Autodesk Fusion 360 part; units mm, degrees
note: some values were not read from the file. Set by a fixed rule: which sketch regions a step uses.
(part 3 of 4)
sketch "Sketch25" plane through (0, 0, 52.9247) normal (0, 0, 1) x (0, -1, 0)
  line L0 (-28.5, -58) -> (-28.5, -55)
  line L1 (-28.5, -58) -> (-25.5, -58)
  line L2 (-25.5, -58) -> (-25.5, -55)
  line L3 (-28.5, -55) -> (-33.0505, -55)
  line L4 (-25.5, -55) -> (-20.9495, -55)
  line L5 (-25.5, 81) -> (-28.5, 81)
  line L6 (-28.5, 81) -> (-28.5, 84)
  line L7 (-25.5, 81) -> (-25.5, 84)
  line L8 (-20.9495, 84) -> (-25.5, 84)
  line L9 (-28.5, 84) -> (-33.0505, 84)
  line L10 (-25.5, 43) -> (-28.5, 43)
  line L11 (-25.5, 46) -> (-28.5, 46)
  line L12 (-25.5, 43) -> (-25.5, 46)
  line L13 (-28.5, 46) -> (-28.5, 43)
  line L14 (-28.5, 56) -> (-25.5, 56)
  line L15 (-25.5, 56) -> (-25.5, 59)
  line L16 (-25.5, 59) -> (-28.5, 59)
  line L17 (-28.5, 59) -> (-28.5, 56)
  line L18 (-23.9495, 52.5) -> (-23.9495, 49.5)
  line L19 (-23.9495, 49.5) -> (-20.9495, 49.5)
  line L20 (-23.9495, 52.5) -> (-20.9495, 52.5)
  line L21 (-20.9495, -55) -> (-20.9495, 49.5)
  line L22 (-20.9495, 52.5) -> (-20.9495, 84)
  line L23 (-30.0505, 52.5) -> (-33.0505, 52.5)
  line L24 (-30.0505, 52.5) -> (-30.0505, 49.5)
  line L25 (-30.0505, 49.5) -> (-33.0505, 49.5)
  line L26 (-33.0505, -55) -> (-33.0505, 49.5)
  line L27 (-33.0505, 52.5) -> (-33.0505, 84)
  dimension "d397" = 139
  dimension "d398" = 139
  dimension "d432" = 12.1009
  dimension "d437" = 3
  dimension "d457" = 1.5505
  constraint coincident L0.end L3.start
  constraint perpendicular L0 L3
  constraint coincident L2.end L4.start
  constraint perpendicular L2 L4
  constraint perpendicular L3 L26
  constraint perpendicular L4 L21
  constraint horizontal L5
  constraint coincident L6.end L8
  constraint perpendicular L6 L8
  constraint perpendicular L7 L8
  constraint collinear L8 L9
  constraint horizontal L10
  constraint horizontal L11
  constraint perpendicular L11 L12
  constraint perpendicular L10 L13
  constraint perpendicular L14 L15
  constraint perpendicular L15 L16
  constraint collinear L21 L22
  constraint collinear L26 L27
  measures "d397" distance of L3.end L9.end
  measures "d398" distance of L4.end L8.start
  measures "d432" distance of L21 L26
  measures "d437" distance of L14.start L14.end
  measures "d457" horizontal distance of L14.end L18.start
extrude "Extrude53" add sketch "Sketch25" along normal blind 3 separate body makes body 53
ref_plane "WorkPlane25" through (81, 49.5, 28.7322) normal (1, 0, 0) x (0, 0, -1)
sketch "Sketch26" plane through (81, 0, 0) normal (1, 0, 0) x (0, 0, -1)
  line L0 (-46.9393, 8.4749) -> (-49.0607, 6.3536)
  line L1 (-49.0607, 6.3536) -> (-51.182, 8.4749)
  line L2 (-49.0607, 10.5962) -> (-51.182, 8.4749)
  line L3 (-49.0607, 10.5962) -> (-51.5355, 13.0711)
  line L4 (-51.9697, 15.5331) -> (-54.9241, 15.0121)
  line L5 (-54.9241, 15.0121) -> (-55.445, 17.9666)
  line L6 (-52.4906, 18.4875) -> (-55.445, 17.9666)
  line L7 (-52.9247, 20.9495) -> (-52.9247, 25.5)
  line L8 (-52.9247, 25.5) -> (-55.9247, 25.5)
  line L9 (-55.9247, 25.5) -> (-55.9247, 28.5)
  line L10 (-52.9247, 28.5) -> (-55.9247, 28.5)
  line L11 (-52.9247, 28.5) -> (-52.9247, 33.0505)
  line L12 (-52.4906, 35.5125) -> (-55.445, 36.0334)
  line L13 (-55.445, 36.0334) -> (-54.9241, 38.9879)
  line L14 (-51.9697, 38.4669) -> (-54.9241, 38.9879)
  line L15 (-51.5355, 40.9289) -> (-49.0607, 43.4038)
  line L16 (-49.0607, 43.4038) -> (-51.182, 45.5251)
  line L17 (-51.182, 45.5251) -> (-49.0607, 47.6464)
  line L18 (-46.9393, 45.5251) -> (-49.0607, 47.6464)
  line L19 (-44.4645, 6) -> (-30.2322, 6)
  line L20 (-30.2322, 6) -> (-30.2322, 3)
  line L21 (-27.2322, 3) -> (-30.2322, 3)
  line L22 (-27.2322, 6) -> (-27.2322, 3)
  line L23 (-27.2322, 6) -> (-13, 6)
  line L24 (-10, 25.5) -> (-13, 25.5)
  line L25 (-10, 28.5) -> (-10, 25.5)
  line L26 (-10, 28.5) -> (-13, 28.5)
  line L27 (-27.2322, 48) -> (-27.2322, 51)
  line L28 (-30.2322, 51) -> (-27.2322, 51)
  line L29 (-30.2322, 48) -> (-30.2322, 51)
  line L30 (-44.4645, 48) -> (-30.2322, 48)
  line L31 (-27.2322, 48) -> (-13, 48)
  line L32 (-13, 6) -> (-13, 25.5)
  line L33 (-13, 28.5) -> (-13, 48)
  line L34 (-44.4645, 6) -> (-46.9393, 8.4749)
  line L35 (-51.5355, 13.0711) -> (-51.9697, 15.5331)
  line L36 (-52.4906, 18.4875) -> (-52.9247, 20.9495)
  line L37 (-52.9247, 33.0505) -> (-52.4906, 35.5125)
  line L38 (-51.9697, 38.4669) -> (-51.5355, 40.9289)
  line L39 (-46.9393, 45.5251) -> (-44.4645, 48)
  line L40 (-32.9624, 28.5) -> (-32.9624, 25.5)
  line L41 (-32.9624, 25.5) -> (-35.9624, 25.5)
  line L42 (-32.9624, 28.5) -> (-35.9624, 28.5)
  line L43 (-35.9624, 28.5) -> (-35.9624, 25.5)
  line L44 (-42.4624, 25.5) -> (-42.4624, 28.5)
  line L45 (-42.4624, 25.5) -> (-45.4624, 25.5)
  line L46 (-45.4624, 25.5) -> (-45.4624, 28.5)
  line L47 (-45.4624, 28.5) -> (-42.4624, 28.5)
  dimension "d503" = 3
  dimension "d504" = 3
  dimension "d676" = 3
  dimension "d677" = 3
  constraint coincident L23.end L32.start
  constraint coincident L24.end L32.end
  constraint coincident L26.end L33.start
  constraint coincident L31.end L33.end
  constraint coincident L19.start L34.start
  constraint coincident L0.start L34.end
  constraint coincident L3.end L35.start
  constraint coincident L4.start L35.end
  constraint coincident L6.start L36.start
  constraint coincident L7.start L36.end
  constraint coincident L11.end L37.start
  constraint coincident L12.start L37.end
  constraint coincident L14.start L38.start
  constraint coincident L15.start L38.end
  constraint coincident L18.start L39.start
  constraint coincident L30.start L39.end
  constraint perpendicular L40 L41
  constraint perpendicular L40 L42
  constraint perpendicular L41 L43
  constraint vertical L44
  constraint perpendicular L44 L45
  constraint perpendicular L45 L46
  measures "d503" distance of L40.end L41.end
  measures "d504" distance of L40.start L42.end
  measures "d676" distance of L44.start L45.end
  measures "d677" distance of L45.end L46.end
extrude "Extrude54" add sketch "Sketch26" along normal blind 3 separate body makes body 54
ref_plane "WorkPlane26" through (84, 27, 32.9624) normal (1, 0, 0) x (0, 0, -1)
sketch "Sketch27" plane through (84, 0, 0) normal (1, 0, 0) x (0, 0, -1)
  line L0 (-35.9624, 28.5) -> (-32.9624, 28.5)
  line L1 (-35.9624, 25.5) -> (-32.9624, 25.5)
  line L2 (-32.9624, 25.5) -> (-32.9624, 28.5)
  line L3 (-35.9624, 28.5) -> (-35.9624, 25.5)
  circle A0 centre (-34.4812, 27) radius 21.4812
  line L4 (-42.4812, 25.5) -> (-42.4812, 28.5)
  line L5 (-42.4812, 25.5) -> (-45.4812, 25.5)
  line L6 (-45.4812, 25.5) -> (-45.4812, 28.5)
  line L7 (-45.4812, 28.5) -> (-42.4812, 28.5)
  dimension "d500" = 3
  dimension "d672" = 3
  dimension "d673" = 3
  dimension "d674" = 3
  constraint horizontal L0
  constraint perpendicular L0 L2
  constraint vertical L4
  constraint perpendicular L4 L5
  constraint perpendicular L5 L6
  measures "d500" distance of L0
  measures "d672" distance of L4.start L4.end
  measures "d673" distance of L4.start L5.end
  measures "d674" distance of L5.end L6.end
extrude "Extrude55" add sketch "Sketch27" along normal blind 3 separate body makes body 55
ref_plane "WorkPlane27" through (87, 27, 34.4812) normal (1, 0, 0) x (0, 0, -1)
sketch "Sketch28" plane through (87, 0, 0) normal (1, 0, 0) x (0, 0, -1)
  line L0 (-35.9624, 25.5) -> (-35.9624, 28.5)
  line L1 (-35.9624, 28.5) -> (-32.9624, 28.5)
  line L2 (-32.9624, 28.5) -> (-32.9624, 25.5)
  line L3 (-32.9624, 25.5) -> (-35.9624, 25.5)
  circle A0 centre (-34.4812, 27) radius 19.481
  line L4 (-42.4812, 25.5) -> (-42.4812, 28.5)
  line L5 (-42.4812, 25.5) -> (-45.4812, 25.5)
  line L6 (-45.4812, 25.5) -> (-45.4812, 28.5)
  line L7 (-45.4812, 28.5) -> (-42.4812, 28.5)
  line L8 (-42.4812, 28.5) -> (-42.4812, 25.5)
  line L9 (-42.4812, 25.5) -> (-45.4812, 25.5)
  line L10 (-45.4812, 25.5) -> (-45.4812, 28.5)
  line L11 (-45.4812, 28.5) -> (-42.4812, 28.5)
  dimension "d501" = 38.962
  dimension "d669" = 3
  dimension "d670" = 3
  constraint vertical L4
  constraint perpendicular L4 L5
  constraint perpendicular L5 L6
  measures "d501" diameter of A0
  measures "d669" distance of L4.start L5.end
  measures "d670" distance of L5.end L6.end
extrude "Extrude56" add sketch "Sketch28" along normal blind 3 separate body makes body 56
ref_plane "WorkPlane28" through (90, 27, 34.4812) normal (1, 0, 0) x (0, 0, -1)
sketch "Sketch29" plane through (90, 0, 0) normal (1, 0, 0) x (0, 0, -1)
  line L0 (-32.9624, 28.5) -> (-32.9624, 25.5)
  line L1 (-32.9624, 25.5) -> (-35.9624, 25.5)
  line L2 (-35.9624, 25.5) -> (-35.9624, 28.5)
  line L3 (-35.9624, 28.5) -> (-32.9624, 28.5)
  circle A0 centre (-34.4812, 27) radius 6
  line L4 (-42.4812, 28.5) -> (-42.4812, 25.5)
  line L5 (-42.4812, 25.5) -> (-45.4812, 25.5)
  line L6 (-45.4812, 25.5) -> (-45.4812, 28.5)
  line L7 (-45.4812, 28.5) -> (-42.4812, 28.5)
  dimension "d502" = 12
  measures "d502" diameter of A0
extrude "Extrude57" add sketch "Sketch29" along normal blind 3 separate body contours A0 makes body 57
ref_plane "WorkPlane29" through (51, 23.9495, 54.4247) normal (0, -1, 0) x (1, 0, 0)
sketch "Sketch30" plane through (0, 23.9495, 0) normal (0, -1, 0) x (1, 0, 0)
  line L0 (52.5, 52.9247) -> (49.5, 52.9247)
  line L1 (49.5, 52.9247) -> (49.5, 55.9247)
  line L2 (52.5, 52.9247) -> (52.5, 55.9247)
  line L3 (52.5, 55.9247) -> (59, 55.9247)
  line L4 (49.5, 55.9247) -> (43, 55.9247)
  line L5 (43, 55.9247) -> (43, 69.4247)
  line L6 (59, 55.9247) -> (59, 69.4247)
  line L7 (43, 69.4247) -> (46, 69.4247)
  line L8 (46, 69.4247) -> (46, 72.4247)
  line L9 (46, 72.4247) -> (43, 72.4247)
  line L10 (43, 72.4247) -> (43, 85.9247)
  line L11 (59, 69.4247) -> (56, 69.4247)
  line L12 (56, 69.4247) -> (56, 72.4247)
  line L13 (56, 72.4247) -> (59, 72.4247)
  line L14 (59, 72.4247) -> (59, 85.9247)
  line L15 (59, 85.9247) -> (43, 85.9247)
  dimension "d449" = 6.5
  dimension "d450" = 6.5
  dimension "d451" = 13.5
  dimension "d452" = 13.5
  dimension "d453" = 3
  dimension "d454" = 13.5
  dimension "d455" = 3
  dimension "d456" = 13.5
  constraint coincident L2.end L3.start
  constraint perpendicular L2 L3
  constraint coincident L1.end L4.start
  constraint perpendicular L1 L4
  constraint perpendicular L4 L5
  constraint perpendicular L3 L6
  constraint perpendicular L5 L7
  constraint perpendicular L7 L8
  constraint perpendicular L8 L9
  constraint perpendicular L9 L10
  constraint perpendicular L6 L11
  constraint perpendicular L11 L12
  constraint perpendicular L12 L13
  constraint perpendicular L13 L14
  measures "d449" distance of L1.end L4.end
  measures "d450" distance of L2.end L3.end
  measures "d451" distance of L4.end L5.end
  measures "d452" distance of L3.end L6.end
  measures "d453" distance of L7.end L8.end
  measures "d454" distance of L9.end L10.end
  measures "d455" distance of L11.end L12.end
  measures "d456" distance of L13.end L14.end
extrude "Extrude58" add sketch "Sketch30" along normal blind 3 separate body makes body 58
ref_plane "WorkPlane30" through (51, 30.0505, 54.4247) normal (0, 1, 0) x (-1, 0, 0)
sketch "Sketch31" plane through (0, 30.0505, 0) normal (0, 1, 0) x (-1, 0, 0)
  line L0 (-52.5, 55.9247) -> (-52.5, 52.9247)
  line L1 (-52.5, 52.9247) -> (-49.5, 52.9247)
  line L2 (-49.5, 52.9247) -> (-49.5, 55.9247)
  line L3 (-49.5, 55.9247) -> (-43, 55.9247)
  line L4 (-59, 55.9247) -> (-52.5, 55.9247)
  line L5 (-43, 55.9247) -> (-43, 69.4247)
  line L6 (-43, 69.4247) -> (-46, 69.4247)
  line L7 (-46, 69.4247) -> (-46, 72.4247)
  line L8 (-46, 72.4247) -> (-43, 72.4247)
  line L9 (-43, 72.4247) -> (-43, 85.9247)
  line L10 (-43, 85.9247) -> (-59, 85.9247)
  line L11 (-59, 85.9247) -> (-59, 72.4247)
  line L12 (-59, 72.4247) -> (-56, 72.4247)
  line L13 (-56, 72.4247) -> (-56, 69.4247)
  line L14 (-56, 69.4247) -> (-59, 69.4247)
  line L15 (-59, 69.4247) -> (-59, 55.9247)
extrude "Extrude59" add sketch "Sketch31" along normal blind 3 separate body makes body 59
ref_plane "WorkPlane31" through (56, 27, 54.4247) normal (1, 0, 0) x (0, 1, 0)
sketch "Sketch32" plane through (56, 0, 0) normal (1, 0, 0) x (0, 1, 0)
  line L0 (20.9495, 69.4247) -> (20.9495, 72.4247)
  line L1 (23.9495, 69.4247) -> (20.9495, 69.4247)
  line L2 (23.9495, 55.9247) -> (23.9495, 69.4247)
  line L3 (30.0505, 69.4247) -> (30.0505, 55.9247)
  line L4 (30.0505, 69.4247) -> (33.0505, 69.4247)
  line L5 (33.0505, 72.4247) -> (33.0505, 69.4247)
  line L6 (30.0505, 72.4247) -> (33.0505, 72.4247)
  line L7 (23.9495, 72.4247) -> (23.9495, 85.9247)
  line L8 (23.9495, 72.4247) -> (20.9495, 72.4247)
  line L9 (30.0505, 85.9247) -> (30.0505, 72.4247)
  line L10 (28.5, 52.9247) -> (28.5, 55.9247)
  line L11 (25.5, 52.9247) -> (28.5, 52.9247)
  line L12 (25.5, 52.9247) -> (25.5, 55.9247)
  line L13 (23.9495, 55.9247) -> (25.5, 55.9247)
  line L14 (28.5, 55.9247) -> (30.0505, 55.9247)
  line L15 (23.9495, 85.9247) -> (30.0505, 85.9247)
  constraint coincident L2.start L13.start
  constraint coincident L12.end L13.end
  constraint coincident L10.end L14.start
  constraint coincident L3.end L14.end
  constraint coincident L7.end L15.start
  constraint coincident L9.start L15.end
extrude "Extrude60" add sketch "Sketch32" along normal blind 3 separate body makes body 60
ref_plane "WorkPlane32" through (46, 27, 54.4247) normal (-1, 0, 0) x (0, -1, 0)
sketch "Sketch33" plane through (46, 0, 0) normal (-1, 0, 0) x (0, -1, 0)
  line L0 (-30.0505, 69.4247) -> (-33.0505, 69.4247)
  line L1 (-33.0505, 69.4247) -> (-33.0505, 72.4247)
  line L2 (-30.0505, 72.4247) -> (-33.0505, 72.4247)
  line L3 (-20.9495, 72.4247) -> (-20.9495, 69.4247)
  line L4 (-23.9495, 72.4247) -> (-20.9495, 72.4247)
  line L5 (-23.9495, 69.4247) -> (-20.9495, 69.4247)
  line L6 (-28.5, 52.9247) -> (-28.5, 55.9247)
  line L7 (-28.5, 52.9247) -> (-25.5, 52.9247)
  line L8 (-25.5, 52.9247) -> (-25.5, 55.9247)
  line L9 (-25.5, 55.9247) -> (-23.9495, 55.9247)
  line L10 (-28.5, 55.9247) -> (-30.0505, 55.9247)
  line L11 (-30.0505, 69.4247) -> (-30.0505, 55.9247)
  line L12 (-23.9495, 69.4247) -> (-23.9495, 55.9247)
  line L13 (-30.0505, 72.4247) -> (-30.0505, 85.9247)
  line L14 (-23.9495, 72.4247) -> (-23.9495, 85.9247)
  line L15 (-30.0505, 85.9247) -> (-23.9495, 85.9247)
  dimension "d462" = 1.5505
  dimension "d463" = 1.5505
  dimension "d464" = 13.5
  dimension "d465" = 13.5
  constraint coincident L8.end L9.start
  constraint perpendicular L8 L9
  constraint coincident L6.end L10.start
  constraint perpendicular L6 L10
  constraint coincident L0.start L11.start
  constraint coincident L5.start L12.start
  constraint coincident L2.start L13.start
  constraint perpendicular L2 L13
  constraint coincident L4.start L14.start
  constraint perpendicular L4 L14
  measures "d462" distance of L8.end L9.end
  measures "d463" distance of L6.end L10.end
  measures "d464" distance of L2.start L13.end
  measures "d465" distance of L4.start L14.end
extrude "Extrude61" add sketch "Sketch33" along normal blind 3 separate body makes body 61
ref_plane "WorkPlane33" through (51, 30.0505, 69.4247) normal (0, -1, 0) x (1, 0, 0)
sketch "Sketch34" plane through (0, 30.0505, 0) normal (0, -1, 0) x (1, 0, 0)
  line L0 (46, 55.9247) -> (56, 55.9247)
  line L1 (56, 55.9247) -> (56, 94.9247)
  line L2 (46, 55.9247) -> (46, 94.9247)
  line L3 (56, 94.9247) -> (46, 94.9247)
  point P0 (46, 55.9247)
  point P1 (56, 55.9247)
  dimension "d469" = 39
  dimension "d470" = 39
  constraint coincident P0 L0.start
  constraint coincident P1 L0.end
  constraint perpendicular L0 L1
  constraint perpendicular L0 L2
  measures "d469" distance of P1 L1.end
  measures "d470" distance of P0 L2.end
extrude "Extrude62" add sketch "Sketch34" along normal blind 3 separate body makes body 62
ref_plane "WorkPlane34" through (51, 27.0505, 75.4247) normal (0, -1, 0) x (0, 0, -1)
sketch "Sketch35" plane through (0, 27.0505, 0) normal (0, -1, 0) x (0, 0, -1)
  line L0 (-55.9247, 46) -> (-55.9247, 56)
  line L1 (-55.9247, 56) -> (-94.9247, 56)
  line L2 (-94.9247, 56) -> (-94.9247, 46)
  line L3 (-94.9247, 46) -> (-55.9247, 46)
extrude "Extrude63" add sketch "Sketch35" along normal blind 3 separate body makes body 63
ref_plane "WorkPlane35" through (51, 22.4495, 85.9247) normal (0, 0, 1) x (-1, 0, 0)
sketch "Sketch36" plane through (0, 0, 85.9247) normal (0, 0, 1) x (-1, 0, 0)
  line L0 (-56, -24.0505) -> (-46, -24.0505)
  line L1 (-46, -24.0505) -> (-46, -30.0505)
  line L2 (-46, -30.0505) -> (-56, -30.0505)
  line L3 (-56, -30.0505) -> (-56, -24.0505)
  line L4 (-63, -16.9495) -> (-38.8991, -16.9495)
  line L5 (-38.8991, -16.9495) -> (-38.8991, -37.0505)
  line L6 (-38.8991, -37.0505) -> (-63, -37.0505)
  line L7 (-63, -16.9495) -> (-63, -37.0505)
  point P0 (-56, -30.0505)
  point P1 (-56, -24.0505)
  point P2 (-46, -24.0505)
  point P3 (-46, -30.0505)
  point P4 (-63, -37.0505)
  dimension "d479" = 20.1009
  dimension "d480" = 24.1009
  dimension "d481" = 20.1009
  dimension "d483" = 24.1009
  constraint coincident P1 L0.start
  constraint coincident P2 L0.end
  constraint coincident P3 L1.end
  constraint coincident P0 L2.end
  constraint perpendicular L4 L5
  constraint coincident P4 L6.end
  measures "d479" distance of L4.start P4
  measures "d480" distance of L4.start L4.end
  measures "d481" distance of L4.end L5.end
  measures "d483" distance of L5.end P4
extrude "Extrude64" add sketch "Sketch36" along normal blind 3 separate body makes body 64
ref_plane "WorkPlane36" through (50.9495, 27, 88.9247) normal (0, 0, 1) x (1, 0, 0)
sketch "Sketch37" plane through (0, 0, 88.9247) normal (0, 0, 1) x (1, 0, 0)
  line L0 (46, 30.0505) -> (56, 30.0505)
  line L1 (56, 30.0505) -> (56, 24.0505)
  line L2 (56, 24.0505) -> (46, 24.0505)
  line L3 (46, 24.0505) -> (46, 30.0505)
  line L4 (38.8991, 16.9495) -> (63, 16.9495)
  line L5 (63, 16.9495) -> (63, 37.0505)
  line L6 (63, 37.0505) -> (38.8991, 37.0505)
  line L7 (38.8991, 37.0505) -> (38.8991, 16.9495)
extrude "Extrude65" add sketch "Sketch37" along normal blind 3 separate body makes body 65
ref_plane "WorkPlane37" through (50.9495, 27, 91.9247) normal (0, 0, 1) x (1, 0, 0)
sketch "Sketch38" plane through (0, 0, 91.9247) normal (0, 0, 1) x (1, 0, 0)
  line L0 (56, 24.0505) -> (46, 24.0505)
  line L1 (46, 24.0505) -> (46, 30.0505)
  line L2 (46, 30.0505) -> (56, 30.0505)
  line L3 (56, 30.0505) -> (56, 24.0505)
  line L4 (38.8991, 37.0505) -> (38.8991, 16.9495)
  line L5 (38.8991, 16.9495) -> (63, 16.9495)
  line L6 (63, 16.9495) -> (63, 37.0505)
  line L7 (63, 37.0505) -> (38.8991, 37.0505)
extrude "Extrude66" add sketch "Sketch38" along normal blind 3 separate body makes body 66
ref_plane "WorkPlane38" through (87.0475, -8.5221, 11.5) normal (0.643192, -0.765705, 0) x (0.765705, 0.643192, 0)
sketch "Sketch39" plane through (40.2083, -47.867, 0) normal (0.643192, -0.765705, 0) x (0.765705, 0.643192, 0)
  line L0 (59.6713, 10) -> (59.6713, 13)
  line L1 (59.6713, 13) -> (62.6713, 13)
  line L2 (62.6713, 10) -> (89.821, 10)
  line L3 (62.6713, 10) -> (62.6713, 13)
  line L4 (89.821, 10) -> (89.821, 13)
  line L5 (89.821, 13) -> (92.821, 13)
  line L6 (92.821, 10) -> (111.9706, 10)
  line L7 (111.9706, 10) -> (111.9706, 13)
  line L8 (111.9706, 13) -> (114.9706, 13)
  line L9 (92.821, 10) -> (92.821, 13)
  line L10 (56.6713, 8) -> (56.6713, -10)
  line L11 (112.9703, -10) -> (112.9703, 8)
  line L12 (59.6344, 8) -> (59.6344, -10)
  line L13 (62.5975, 8) -> (62.5975, -10)
  line L14 (65.5606, 8) -> (65.5606, -10)
  line L15 (68.5238, 8) -> (68.5238, -10)
  line L16 (71.4869, 8) -> (71.4869, -10)
  line L17 (74.45, 8) -> (74.45, -10)
  line L18 (77.4131, 8) -> (77.4131, -10)
  line L19 (80.3762, 8) -> (80.3762, -10)
  line L20 (83.3393, 8) -> (83.3393, -10)
  line L21 (86.3024, 8) -> (86.3024, -10)
  line L22 (89.2655, 8) -> (89.2655, -10)
  line L23 (92.2286, 8) -> (92.2286, -10)
  line L24 (95.1917, 8) -> (95.1917, -10)
  line L25 (98.1548, 8) -> (98.1548, -10)
  line L26 (101.1179, 8) -> (101.1179, -10)
  line L27 (104.081, 8) -> (104.081, -10)
  line L28 (107.0441, 8) -> (107.0441, -10)
  line L29 (110.0072, 8) -> (110.0072, -10)
  line L30 (112.9703, 8) -> (112.9703, -10)
  line L31 (56.6713, 8) -> (59.6344, 8)
  line L32 (62.5975, 8) -> (65.5606, 8)
  line L33 (68.5238, 8) -> (71.4869, 8)
  line L34 (74.45, 8) -> (77.4131, 8)
  line L35 (80.3762, 8) -> (83.3393, 8)
  line L36 (86.3024, 8) -> (89.2655, 8)
  line L37 (92.2286, 8) -> (95.1917, 8)
  line L38 (98.1548, 8) -> (101.1179, 8)
  line L39 (104.081, 8) -> (107.0441, 8)
  line L40 (110.0072, 8) -> (112.9703, 8)
  line L41 (115.9706, 10) -> (115.9706, -12)
  line L42 (114.9706, 13) -> (114.9706, 10)
  line L43 (114.9706, 10) -> (115.9706, 10)
  line L44 (53.6713, 10) -> (53.6713, -12)
  line L45 (59.6713, 10) -> (53.6713, 10)
  line L46 (59.6344, -10) -> (56.6713, -10)
  line L47 (65.5606, -10) -> (62.5975, -10)
  line L48 (71.4869, -10) -> (68.5238, -10)
  line L49 (77.4131, -10) -> (74.45, -10)
  line L50 (83.3393, -10) -> (80.3762, -10)
  line L51 (89.2655, -10) -> (86.3024, -10)
  line L52 (95.1917, -10) -> (92.2286, -10)
  line L53 (101.1179, -10) -> (98.1548, -10)
  line L54 (112.9703, -10) -> (110.0072, -10)
  line L55 (107.0441, -10) -> (104.081, -10)
  line L56 (115.9706, -12) -> (53.6713, -12)
  dimension "d547" = 56.299
  constraint vertical L10
  constraint collinear L31 L32
  constraint collinear L32 L33
  constraint collinear L33 L34
  constraint collinear L34 L35
  constraint collinear L35 L36
  constraint collinear L36 L37
  constraint collinear L37 L38
  constraint collinear L38 L39
  constraint collinear L39 L40
  constraint coincident L8.end L42.start
  constraint perpendicular L8 L42
  constraint perpendicular L41 L43
  constraint coincident L0.start L45.start
  constraint perpendicular L44 L45
  constraint coincident L12.end L54
  constraint collinear L46 L54
  constraint coincident L14.end L54
  constraint collinear L47 L54
  constraint coincident L16.end L54
  constraint collinear L48 L54
  constraint coincident L18.end L54
  constraint collinear L49 L54
  constraint coincident L20.end L54
  constraint collinear L50 L54
  constraint coincident L22.end L54
  constraint collinear L51 L54
  constraint coincident L24.end L54
  constraint collinear L52 L54
  constraint coincident L26.end L54
  constraint collinear L53 L54
  constraint coincident L28.end L54
  constraint collinear L54 L55
  measures "d547" distance of L10.start L11.end
extrude "Extrude67" add sketch "Sketch39" along normal blind 3 separate body makes body 67
ref_plane "WorkPlane39" through (87.0475, 62.5221, 11.5) normal (0.643192, 0.765705, 0) x (-0.765705, 0.643192, 0)
sketch "Sketch40" plane through (66.8031, 79.5275, 0) normal (0.643192, 0.765705, 0) x (-0.765705, 0.643192, 0)
  line L0 (-27.939, 10) -> (-27.939, 13)
  line L1 (-27.939, 13) -> (-24.939, 13)
  line L2 (-27.939, 10) -> (-55.0886, 10)
  line L3 (-24.939, 10) -> (-24.939, 13)
  line L4 (-55.0886, 10) -> (-55.0886, 13)
  line L5 (-58.0886, 13) -> (-55.0886, 13)
  line L6 (-58.0886, 10) -> (-77.2383, 10)
  line L7 (-77.2383, 10) -> (-77.2383, 13)
  line L8 (-80.2383, 13) -> (-77.2383, 13)
  line L9 (-58.0886, 10) -> (-58.0886, 13)
  line L10 (-80.2383, 10) -> (-80.2383, 13)
  line L11 (-21.939, 8) -> (-21.939, -10)
  line L12 (-78.2383, 8) -> (-78.2383, -10)
  line L13 (-24.9021, 8) -> (-24.9021, -10)
  line L14 (-27.8652, 8) -> (-27.8652, -10)
  line L15 (-30.8283, 8) -> (-30.8283, -10)
  line L16 (-33.7914, 8) -> (-33.7914, -10)
  line L17 (-36.7546, 8) -> (-36.7546, -10)
  line L18 (-39.7177, 8) -> (-39.7177, -10)
  line L19 (-42.6808, 8) -> (-42.6808, -10)
  line L20 (-45.6439, 8) -> (-45.6439, -10)
  line L21 (-48.6071, 8) -> (-48.6071, -10)
  line L22 (-51.5702, 8) -> (-51.5702, -10)
  line L23 (-54.5333, 8) -> (-54.5333, -10)
  line L24 (-57.4964, 8) -> (-57.4964, -10)
  line L25 (-60.4595, 8) -> (-60.4595, -10)
  line L26 (-63.4227, 8) -> (-63.4227, -10)
  line L27 (-66.3858, 8) -> (-66.3858, -10)
  line L28 (-69.3489, 8) -> (-69.3489, -10)
  line L29 (-72.312, 8) -> (-72.312, -10)
  line L30 (-75.2751, 8) -> (-75.2751, -10)
  line L31 (-78.2383, 8) -> (-78.2383, -10)
  line L32 (-21.939, 8) -> (-24.9021, 8)
  line L33 (-27.8652, 8) -> (-30.8283, 8)
  line L34 (-33.7914, 8) -> (-36.7546, 8)
  line L35 (-39.7177, 8) -> (-42.6808, 8)
  line L36 (-45.6439, 8) -> (-48.6071, 8)
  line L37 (-51.5702, 8) -> (-54.5333, 8)
  line L38 (-57.4964, 8) -> (-60.4595, 8)
  line L39 (-63.4227, 8) -> (-66.3858, 8)
  line L40 (-69.3489, 8) -> (-72.312, 8)
  line L41 (-75.2751, 8) -> (-78.2383, 8)
  line L42 (-81.2383, 10) -> (-81.2383, -12)
  line L43 (-81.2383, 10) -> (-80.2383, 10)
  line L44 (-18.939, 10) -> (-18.939, -12)
  line L45 (-24.939, 10) -> (-18.939, 10)
  line L46 (-24.9021, -10) -> (-21.939, -10)
  line L47 (-30.8283, -10) -> (-27.8652, -10)
  line L48 (-36.7546, -10) -> (-33.7914, -10)
  line L49 (-42.6808, -10) -> (-39.7177, -10)
  line L50 (-48.6071, -10) -> (-45.6439, -10)
  line L51 (-54.5333, -10) -> (-51.5702, -10)
  line L52 (-60.4595, -10) -> (-57.4964, -10)
  line L53 (-66.3858, -10) -> (-63.4227, -10)
  line L54 (-72.312, -10) -> (-69.3489, -10)
  line L55 (-78.2383, -10) -> (-75.2751, -10)
  line L56 (-81.2383, -12) -> (-18.939, -12)
  constraint perpendicular L11 L32
  constraint collinear L32 L33
  constraint collinear L33 L34
  constraint collinear L34 L35
  constraint collinear L35 L36
  constraint collinear L36 L37
  constraint collinear L37 L38
  constraint collinear L38 L39
  constraint collinear L39 L40
  constraint collinear L40 L41
  constraint coincident L10.start L43.end
  constraint perpendicular L10 L43
  constraint coincident L3.start L45.start
  constraint perpendicular L44 L45
extrude "Extrude68" add sketch "Sketch40" along normal blind 3 separate body makes body 68
ref_plane "WorkPlane40" through (90, 27, 34.4812) normal (1, 0, 0) x (0, 0, -1)
sketch "Sketch41" plane through (90, 0, 0) normal (1, 0, 0) x (0, 0, -1)
  arc A0 (-34.4812, 34) -> (-34.4812, 20) centre (-34.4812, 27) ccw
  arc A1 (-34.4812, 39) -> (-34.4812, 15) centre (-34.4812, 27) ccw
  line L0 (-34.4812, 34) -> (-34.4812, 39)
  line L1 (-34.4812, 20) -> (-34.4812, 15)
  line L2 (-45.4812, 25.5) -> (-42.4812, 25.5)
  line L3 (-42.4812, 28.5) -> (-45.4812, 28.5)
  line L4 (-45.4812, 25.5) -> (-45.4812, 28.5)
  line L5 (-42.4812, 28.5) -> (-42.4812, 25.5)
  dimension "d594" = 3
  dimension "d595" = 3
  constraint vertical L0
  constraint parallel L0 L1
  constraint parallel L4 L5
  measures "d594" distance of L2.start L2.end
  measures "d595" distance of L3.start L3.end
extrude "Extrude69" add sketch "Sketch41" along normal blind 3 separate body makes body 69
ref_plane "WorkPlane41" through (93, 27, 40.4812) normal (1, 0, 0) x (0, 0, -1)
sketch "Sketch42" plane through (93, 0, 0) normal (1, 0, 0) x (0, 0, -1)
  line L0 (-42.4812, 25.5) -> (-45.4812, 25.5)
  line L1 (-45.4812, 25.5) -> (-45.4812, 28.5)
  line L2 (-45.4812, 28.5) -> (-42.4812, 28.5)
  line L3 (-42.4812, 28.5) -> (-42.4812, 25.5)
  line L4 (-34.4812, 34) -> (-34.4812, 39)
  arc A0 (-34.4812, 39) -> (-34.4812, 15) centre (-34.4812, 27) ccw
  line L5 (-34.4812, 15) -> (-34.4812, 20)
  arc A1 (-34.4812, 34) -> (-34.4812, 20) centre (-34.4812, 27) ccw
extrude "Extrude70" add sketch "Sketch42" along normal blind 3 separate body makes body 70
ref_plane "WorkPlane42" through (96, 27, 40.4812) normal (1, 0, 0) x (0, 0, -1)
sketch "Sketch43" plane through (96, 0, 0) normal (1, 0, 0) x (0, 0, -1)
  line L0 (-45.4812, 28.5) -> (-42.4812, 28.5)
  line L1 (-42.4812, 28.5) -> (-42.4812, 25.5)
  line L2 (-42.4812, 25.5) -> (-45.4812, 25.5)
  line L3 (-45.4812, 25.5) -> (-45.4812, 28.5)
  arc A0 (-34.4812, 39) -> (-34.4812, 15) centre (-34.4812, 27) ccw
  line L4 (-34.4812, 15) -> (-34.4812, 20)
  arc A1 (-34.4812, 34) -> (-34.4812, 20) centre (-34.4812, 27) ccw
  line L5 (-34.4812, 34) -> (-34.4812, 39)
extrude "Extrude71" add sketch "Sketch43" along normal blind 3 separate body makes body 71
ref_plane "WorkPlane43" through (60, -7.5, 15.6471) normal (1, 0, 0) x (0, 0, 1)
sketch "Sketch44" plane through (60, 0, 0) normal (1, 0, 0) x (0, 1, 0)
  line L0 (-6, 15) -> (-9, 15)
  line L1 (-9, 15) -> (-9, 16.2941)
  line L2 (-6, 16.2941) -> (-9, 16.2941)
  line L3 (-6, 16.2941) -> (-6, 15)
  line L4 (-14, 11) -> (0, 11)
  line L5 (-14, 20.2941) -> (3, 20.2941)
  line L6 (-14, 11) -> (-14, 20.2941)
  line L7 (6, 15) -> (6, 16.2941)
  line L8 (0, 13) -> (3, 13)
  line L9 (0, 13) -> (0, 11)
  line L10 (3, 16.2941) -> (6, 16.2941)
  line L11 (3, 15) -> (6, 15)
  line L12 (3, 20.2941) -> (3, 16.2941)
  line L13 (3, 15) -> (3, 13)
  point P0 (0, 13)
  constraint perpendicular L3 L4
  constraint perpendicular L5 L6
  constraint coincident P0 L8.start
  constraint perpendicular L4 L9
  constraint perpendicular L7 L10
  constraint perpendicular L7 L11
  constraint perpendicular L11 L12
  constraint collinear L12 L13
extrude "Extrude72" add sketch "Sketch44" along normal blind 3 separate body makes body 72
ref_plane "WorkPlane44" through (63, -4, 15.6471) normal (1, 0, 0) x (0, 0, -1)
sketch "Sketch45" plane through (63, 0, 0) normal (1, 0, 0) x (0, 1, 0)
  line L0 (-9, 16.2941) -> (-6, 16.2941)
  line L1 (-6, 16.2941) -> (-6, 15)
  line L2 (-6, 15) -> (-9, 15)
  line L3 (-9, 15) -> (-9, 16.2941)
  line L4 (6, 15) -> (6, 16.2941)
  line L5 (6, 16.2941) -> (3, 16.2941)
  line L6 (3, 16.2941) -> (3, 20.2941)
  line L7 (3, 20.2941) -> (-14, 20.2941)
  line L8 (-14, 20.2941) -> (-14, 11)
  line L9 (-14, 11) -> (0, 11)
  line L10 (0, 11) -> (0, 13)
  line L11 (0, 13) -> (3, 13)
  line L12 (3, 13) -> (3, 15)
  line L13 (3, 15) -> (6, 15)
extrude "Extrude73" add sketch "Sketch45" along normal blind 3 separate body makes body 73
ref_plane "WorkPlane45" through (66, -4, 15.6471) normal (1, 0, 0) x (0, 0, -1)
sketch "Sketch46" plane through (66, 0, 0) normal (1, 0, 0) x (0, 1, 0)
  line L0 (-6, 15) -> (-9, 15)
  line L1 (-9, 15) -> (-9, 16.2941)
  line L2 (-9, 16.2941) -> (-6, 16.2941)
  line L3 (-6, 16.2941) -> (-6, 15)
  line L4 (3, 15) -> (6, 15)
  line L5 (6, 15) -> (6, 16.2941)
  line L6 (6, 16.2941) -> (3, 16.2941)
  line L7 (3, 16.2941) -> (3, 20.2941)
  line L8 (3, 20.2941) -> (-14, 20.2941)
  line L9 (-14, 20.2941) -> (-14, 11)
  line L10 (-14, 11) -> (0, 11)
  line L11 (0, 11) -> (0, 13)
  line L12 (0, 13) -> (3, 13)
  line L13 (3, 13) -> (3, 15)
extrude "Extrude74" add sketch "Sketch46" along normal blind 3 separate body makes body 74
ref_plane "WorkPlane46" through (69, -4, 15.6471) normal (1, 0, 0) x (0, 0, -1)
sketch "Sketch47" plane through (69, 0, 0) normal (1, 0, 0) x (0, 1, 0)
  line L0 (-9, 16.2941) -> (-6, 16.2941)
  line L1 (-6, 16.2941) -> (-6, 15)
  line L2 (-6, 15) -> (-9, 15)
  line L3 (-9, 15) -> (-9, 16.2941)
  line L4 (3, 13) -> (3, 15)
  line L5 (3, 15) -> (6, 15)
  line L6 (6, 15) -> (6, 16.2941)
  line L7 (6, 16.2941) -> (3, 16.2941)
  line L8 (3, 16.2941) -> (3, 20.2941)
  line L9 (3, 20.2941) -> (-14, 20.2941)
  line L10 (-14, 20.2941) -> (-14, 11)
  line L11 (-14, 11) -> (0, 11)
  line L12 (0, 11) -> (0, 13)
  line L13 (0, 13) -> (3, 13)
extrude "Extrude75" add sketch "Sketch47" along normal blind 3 separate body makes body 75
ref_plane "WorkPlane47" through (72, -4, 15.6471) normal (1, 0, 0) x (0, 0, -1)
sketch "Sketch48" plane through (72, 0, 0) normal (1, 0, 0) x (0, 1, 0)
  line L0 (-6, 15) -> (-9, 15)
  line L1 (-9, 15) -> (-9, 16.2941)
  line L2 (-9, 16.2941) -> (-6, 16.2941)
  line L3 (-6, 16.2941) -> (-6, 15)
  line L4 (0, 13) -> (3, 13)
  line L5 (3, 13) -> (3, 15)
  line L6 (3, 15) -> (6, 15)
  line L7 (6, 15) -> (6, 16.2941)
  line L8 (6, 16.2941) -> (3, 16.2941)
  line L9 (3, 16.2941) -> (3, 20.2941)
  line L10 (3, 20.2941) -> (-14, 20.2941)
  line L11 (-14, 20.2941) -> (-14, 11)
  line L12 (-14, 11) -> (0, 11)
  line L13 (0, 11) -> (0, 13)
extrude "Extrude76" add sketch "Sketch48" along normal blind 3 separate body makes body 76
ref_plane "WorkPlane48" through (75, -4, 15.6471) normal (1, 0, 0) x (0, 0, -1)
sketch "Sketch49" plane through (75, 0, 0) normal (1, 0, 0) x (0, 1, 0)
  line L0 (-9, 16.2941) -> (-6, 16.2941)
  line L1 (-6, 16.2941) -> (-6, 15)
  line L2 (-6, 15) -> (-9, 15)
  line L3 (-9, 15) -> (-9, 16.2941)
  line L4 (0, 11) -> (0, 13)
  line L5 (0, 13) -> (3, 13)
  line L6 (3, 13) -> (3, 15)
  line L7 (3, 15) -> (6, 15)
  line L8 (6, 15) -> (6, 16.2941)
  line L9 (6, 16.2941) -> (3, 16.2941)
  line L10 (3, 16.2941) -> (3, 20.2941)
  line L11 (3, 20.2941) -> (-14, 20.2941)
  line L12 (-14, 20.2941) -> (-14, 11)
  line L13 (-14, 11) -> (0, 11)
extrude "Extrude77" add sketch "Sketch49" along normal blind 3 separate body makes body 77
ref_plane "WorkPlane49" through (78, 61.5, 15.6471) normal (1, 0, 0) x (0, 0, -1)
sketch "Sketch50" plane through (78, 0, 0) normal (1, 0, 0) x (0, 0, -1)
  line L0 (-20.2941, 68) -> (-11, 68)
  line L1 (-11, 68) -> (-11, 54)
  line L2 (-11, 54) -> (-13, 54)
  line L3 (-13, 54) -> (-13, 51)
  line L4 (-13, 51) -> (-15, 51)
  line L5 (-15, 51) -> (-15, 48)
  line L6 (-15, 48) -> (-16.2941, 48)
  line L7 (-16.2941, 48) -> (-16.2941, 51)
  line L8 (-16.2941, 51) -> (-20.2941, 51)
  line L9 (-20.2941, 51) -> (-20.2941, 68)
  line L10 (-15, 60) -> (-15, 63)
  line L11 (-15, 63) -> (-16.2941, 63)
  line L12 (-16.2941, 63) -> (-16.2941, 60)
  line L13 (-16.2941, 60) -> (-15, 60)
extrude "Extrude78" add sketch "Sketch50" against normal blind 3 separate body makes body 78
ref_plane "WorkPlane50" through (75, 58, 15.6471) normal (-1, 0, 0) x (0, 0, 1)
sketch "Sketch51" plane through (75, 0, 0) normal (-1, 0, 0) x (0, 0, 1)
  line L0 (16.2941, 60) -> (15, 60)
  line L1 (15, 60) -> (15, 63)
  line L2 (15, 63) -> (16.2941, 63)
  line L3 (16.2941, 63) -> (16.2941, 60)
  line L4 (16.2941, 51) -> (20.2941, 51)
  line L5 (20.2941, 51) -> (20.2941, 68)
  line L6 (20.2941, 68) -> (11, 68)
  line L7 (11, 68) -> (11, 54)
  line L8 (11, 54) -> (13, 54)
  line L9 (13, 54) -> (13, 51)
  line L10 (13, 51) -> (15, 51)
  line L11 (15, 51) -> (15, 48)
  line L12 (15, 48) -> (16.2941, 48)
  line L13 (16.2941, 48) -> (16.2941, 51)
extrude "Extrude79" add sketch "Sketch51" along normal blind 3 separate body makes body 79
ref_plane "WorkPlane51" through (72, 58, 15.6471) normal (-1, 0, 0) x (0, 0, 1)
sketch "Sketch52" plane through (72, 0, 0) normal (-1, 0, 0) x (0, 0, 1)
  line L0 (15, 63) -> (16.2941, 63)
  line L1 (16.2941, 63) -> (16.2941, 60)
  line L2 (16.2941, 60) -> (15, 60)
  line L3 (15, 60) -> (15, 63)
  line L4 (16.2941, 48) -> (16.2941, 51)
  line L5 (16.2941, 51) -> (20.2941, 51)
  line L6 (20.2941, 51) -> (20.2941, 68)
  line L7 (20.2941, 68) -> (11, 68)
  line L8 (11, 68) -> (11, 54)
  line L9 (11, 54) -> (13, 54)
  line L10 (13, 54) -> (13, 51)
  line L11 (13, 51) -> (15, 51)
  line L12 (15, 51) -> (15, 48)
  line L13 (15, 48) -> (16.2941, 48)
extrude "Extrude80" add sketch "Sketch52" along normal blind 3 separate body makes body 80
ref_plane "WorkPlane52" through (69, 58, 15.6471) normal (-1, 0, 0) x (0, 0, 1)
sketch "Sketch53" plane through (69, 0, 0) normal (-1, 0, 0) x (0, 0, 1)
sketch "Sketch54" plane through (69, 0, 0) normal (-1, 0, 0) x (0, -1, 0)
  line L0 (-60, 16.2941) -> (-60, 15)
  line L1 (-60, 15) -> (-63, 15)
  line L2 (-63, 15) -> (-63, 16.2941)
  line L3 (-63, 16.2941) -> (-60, 16.2941)
  line L4 (-48, 15) -> (-48, 16.2941)
  line L5 (-48, 16.2941) -> (-51, 16.2941)
  line L6 (-51, 16.2941) -> (-51, 20.2941)
  line L7 (-51, 20.2941) -> (-68, 20.2941)
  line L8 (-68, 20.2941) -> (-68, 11)
  line L9 (-68, 11) -> (-54, 11)
  line L10 (-54, 11) -> (-54, 13)
  line L11 (-54, 13) -> (-51, 13)
  line L12 (-51, 13) -> (-51, 15)
  line L13 (-51, 15) -> (-48, 15)
extrude "Extrude81" add sketch "Sketch54" along normal blind 3 separate body makes body 81
ref_plane "WorkPlane53" through (66, 58, 15.6471) normal (-1, 0, 0) x (0, 0, 1)
sketch "Sketch55" plane through (66, 0, 0) normal (-1, 0, 0) x (0, 0, 1)
  line L0 (15, 63) -> (16.2941, 63)
  line L1 (16.2941, 63) -> (16.2941, 60)
  line L2 (16.2941, 60) -> (15, 60)
  line L3 (15, 60) -> (15, 63)
  line L4 (15, 51) -> (15, 48)
  line L5 (15, 48) -> (16.2941, 48)
  line L6 (16.2941, 48) -> (16.2941, 51)
  line L7 (16.2941, 51) -> (20.2941, 51)
  line L8 (20.2941, 51) -> (20.2941, 68)
  line L9 (20.2941, 68) -> (11, 68)
  line L10 (11, 68) -> (11, 54)
  line L11 (11, 54) -> (13, 54)
  line L12 (13, 54) -> (13, 51)
  line L13 (13, 51) -> (15, 51)
extrude "Extrude82" add sketch "Sketch55" along normal blind 3 separate body makes body 82
ref_plane "WorkPlane54" through (63, 58, 15.6471) normal (-1, 0, 0) x (0, 0, 1)
sketch "Sketch56" plane through (63, 0, 0) normal (-1, 0, 0) x (0, 0, 1)
  line L0 (16.2941, 60) -> (15, 60)
  line L1 (15, 60) -> (15, 63)
  line L2 (15, 63) -> (16.2941, 63)
  line L3 (16.2941, 63) -> (16.2941, 60)
  line L4 (13, 51) -> (15, 51)
  line L5 (15, 51) -> (15, 48)
  line L6 (15, 48) -> (16.2941, 48)
  line L7 (16.2941, 48) -> (16.2941, 51)
  line L8 (16.2941, 51) -> (20.2941, 51)
  line L9 (20.2941, 51) -> (20.2941, 68)
  line L10 (20.2941, 68) -> (11, 68)
  line L11 (11, 68) -> (11, 54)
  line L12 (11, 54) -> (13, 54)
  line L13 (13, 54) -> (13, 51)
extrude "Extrude83" add sketch "Sketch56" along normal blind 3 separate body makes body 83
ref_plane "WorkPlane55" through (71, -9, -1.5) normal (0, -1, 0) x (-1, 0, 0)
sketch "Sketch57" plane through (0, -9, 0) normal (0, -1, 0) x (-1, 0, 0)
  line L0 (82.5, 9) -> (82.5, 3)
  line L1 (82.5, 3) -> (79.5, 3)
  line L2 (79.5, 3) -> (79.5, 9)
  line L3 (79.5, 9) -> (82.5, 9)
  line L4 (62.5, 9) -> (62.5, 3)
  line L5 (62.5, 3) -> (59.5, 3)
  line L6 (59.5, 9) -> (62.5, 9)
  line L7 (59.5, 3) -> (59.5, 9)
  line L8 (36.5, 3) -> (36.5, -3)
  line L9 (33.5, 3) -> (36.5, 3)
  line L10 (33.5, -3) -> (33.5, 3)
  line L11 (36.5, -3) -> (33.5, -3)
  line L12 (1.5, 3) -> (1.5, -3)
  line L13 (1.5, -2.9851) -> (-1.5, -2.9851)
  line L14 (-1.5, -3) -> (-1.5, 3)
  line L15 (-1.5, 3) -> (1.5, 3)
  line L16 (-33.5, 3) -> (-33.5, -3)
  line L17 (-33.5, -2.9851) -> (-36.5, -2.9851)
  line L18 (-36.5, -3) -> (-36.5, 3)
  line L19 (-36.5, 3) -> (-33.5, 3)
  line L20 (-79.5, 9) -> (-79.5, 3)
  line L21 (-82.5, 9) -> (-79.5, 9)
  line L22 (-79.5, 3) -> (-82.5, 3)
  line L23 (-62.5, 9) -> (-59.5, 9)
  line L24 (-59.5, 9) -> (-59.5, 3)
  line L25 (-59.5, 3) -> (-62.5, 3)
  line L26 (-62.5, 3) -> (-62.5, 9)
  line L27 (-82.5, 3) -> (-82.5, 9)
  dimension "d763" = 6
  measures "d763" distance of L16.start L16.end
extrude "Extrude84" add sketch "Sketch57" against normal blind 72 separate body contours L0 L1 L2 L3 makes body 84
extrude "Extrude85" add sketch "Sketch57" against normal blind 72 separate body contours L4 L5 L6 L7 makes body 85
extrude "Extrude86" add sketch "Sketch57" against normal blind 72 separate body contours L8 L9 L10 L11 makes body 86
extrude "Extrude87" add sketch "Sketch57" against normal blind 72 separate body contours L12 L13 L14 L15 makes body 87
extrude "Extrude88" add sketch "Sketch57" against normal blind 72 separate body contours L16 L17 L18 L19 makes body 88
extrude "Extrude89" add sketch "Sketch57" against normal blind 72 separate body contours L23 L24 L25 L26 makes body 89
extrude "Extrude90" add sketch "Sketch57" against normal blind 72 separate body contours L20 L21 L22 L27 makes body 90
ref_plane "WorkPlane56" through (99, 27, 40.4812) normal (1, 0, 0) x (0, 0, -1)
sketch "Sketch58" plane through (99, 0, 0) normal (1, 0, 0) x (0, 0, -1)
  line L0 (-42.4812, 28.5) -> (-42.4812, 25.5)
  line L1 (-42.4812, 25.5) -> (-45.4812, 25.5)
  line L2 (-45.4812, 25.5) -> (-45.4812, 28.5)
  line L3 (-45.4812, 28.5) -> (-42.4812, 28.5)
extrude "Extrude91" add sketch "Sketch58" against normal blind 18 separate body makes body 91
ref_plane "WorkPlane57" through (93, 27, 34.4812) normal (1, 0, 0) x (0, 0, -1)
sketch "Sketch59" plane through (93, 0, 0) normal (1, 0, 0) x (0, 0, -1)
  line L0 (-32.9624, 28.5) -> (-32.9624, 25.5)
  line L1 (-32.9624, 25.5) -> (-35.9624, 25.5)
  line L2 (-35.9624, 25.5) -> (-35.9624, 28.5)
  line L3 (-35.9624, 28.5) -> (-32.9624, 28.5)
extrude "Extrude92" add sketch "Sketch59" against normal blind 12 separate body makes body 92
ref_plane "WorkPlane58" through (18, 27, 10) normal (0, 0, -1) x (-1, 0, 0)
sketch "Sketch60" plane through (0, 0, 10) normal (0, 0, -1) x (-1, 0, 0)
  line L0 (95, 25.5) -> (98, 25.5)
  line L1 (95, 28.5) -> (95, 25.5)
  line L2 (95, 28.5) -> (98, 28.5)
  line L3 (98, 28.5) -> (98, 25.5)
  line L4 (91, 21.5) -> (91, 32.5)
  line L5 (91, 32.5) -> (105.5, 32.5)
  line L6 (91, 21.5) -> (105.5, 21.5)
  arc A0 (111, 27) -> (105.5, 32.5) centre (105.5, 27) ccw
  arc A1 (105.5, 21.5) -> (111, 27) centre (105.5, 27) ccw
  line L7 (108.5, 28.5) -> (108.5, 25.5)
  line L8 (108.5, 28.5) -> (105.5, 28.5)
  line L9 (108.5, 25.5) -> (105.5, 25.5)
  line L10 (105.5, 25.5) -> (105.5, 28.5)
  point P0 (111, 32.5)
  point P1 (111, 21.5)
  dimension "d688" = 11
  dimension "d692" = 20
  dimension "d693" = 20
  dimension "d721" = 5.5
  dimension "d722" = 5.5
  dimension "d725" = 3
  dimension "d726" = 3
  constraint perpendicular L4 L5
  constraint perpendicular L4 L6
  constraint coincident P0 L5
  constraint tangent L5 A0
  constraint coincident P1 L6
  constraint coincident A0.start A1.end
  constraint perpendicular L7 L8
  constraint perpendicular L7 L9
  constraint perpendicular L8 L10
  measures "d688" distance of L4.start L4.end
  measures "d692" distance of L4.end P0
  measures "d693" distance of L4.start P1
  measures "d721" radius of A0
  measures "d722" radius of A1
  measures "d725" distance of L7.start L8.end
  measures "d726" distance of L7.end L9.end
extrude "Extrude93" add sketch "Sketch60" along normal blind 3 separate body makes body 93
ref_plane "WorkPlane59" through (-85, 43.5, 11.5) normal (-1, 0, 0) x (0, -1, 0)
sketch "Sketch61" plane through (-85, 0, 0) normal (-1, 0, 0) x (0, -1, 0)
  line L0 (-45, 10) -> (-45, 13)
  line L1 (-45, 13) -> (-42, 13)
  line L2 (-42, 10) -> (-42, 13)
  line L3 (-12, 13) -> (-9, 13)
  line L4 (-9, 10) -> (-9, 13)
  line L5 (-12, 10) -> (-12, 13)
  line L6 (-45, 10) -> (-51, 10)
  line L7 (-42, 10) -> (-12, 10)
  line L8 (-9, 10) -> (-3, 10)
  line L9 (-3, -10) -> (-51, -10)
  line L10 (-3, -10) -> (-3, -4.5)
  line L11 (-3, -4.5) -> (0, -4.5)
  line L12 (0, -4.5) -> (0, -1.5)
  line L13 (0, -1.5) -> (-3, -1.5)
  line L14 (-3, -1.5) -> (-3, 10)
  line L15 (-51, -10) -> (-51, -7)
  line L16 (-51, -7) -> (-54, -7)
  line L17 (-54, -7) -> (-54, -4)
  line L18 (-54, -4) -> (-51, -4)
  line L19 (-51, -4) -> (-51, 10)
  point P0 (-51, 10)
  point P1 (-3, 10)
  point P2 (-3, -10)
  point P3 (-51, -10)
  point P4 (-51, -5)
  dimension "d710" = 5.5
  dimension "d711" = 3
  dimension "d712" = 3
  constraint coincident L0.start L6.start
  constraint coincident P0 L6.end
  constraint coincident L2.start L7.start
  constraint coincident L5.start L7.end
  constraint coincident L4.start L8.start
  constraint coincident P1 L8.end
  constraint perpendicular L9 L10
  constraint perpendicular L10 L11
  constraint perpendicular L11 L12
  constraint perpendicular L12 L13
  constraint perpendicular L9 L15
  constraint perpendicular L15 L16
  constraint perpendicular L16 L17
  constraint perpendicular L17 L18
  measures "d710" distance of P2 L10.end
  measures "d711" distance of L11.end L12.end
  measures "d712" distance of L16.end L17.end
extrude "Extrude94" add sketch "Sketch61" along normal blind 3 separate body makes body 94
move_body "Move1" bodies 94 to x (1, 0, 0) y (0, 1, 0) z (0, 0, 1) at (0, 0, 9)
move_body "Move2" bodies 94 to x (1, 0, 0) y (0, 1, 0) z (0, 0, 1) at (0, 0, -9)
ref_plane "WorkPlane60" through (87, 52.5, 0) normal (1, 0, 0) x (0, 0, -1)
sketch "Sketch62" plane through (87, 0, 0) normal (1, 0, 0) x (0, 0, -1)
  line L0 (-1.5, 0) -> (-10, 0)
  line L1 (-1.5, 3) -> (-1.5, 0)
  line L2 (1.5, 3) -> (-1.5, 3)
  line L3 (1.5, 3) -> (1.5, 0)
  line L4 (10, 0) -> (1.5, 0)
  line L5 (1.5, 51) -> (-1.5, 51)
  line L6 (-1.5, 51) -> (-1.5, 54)
  line L7 (1.5, 51) -> (1.5, 54)
  line L8 (1.5, 54) -> (10, 54)
  line L9 (-10, 54) -> (-1.5, 54)
  line L10 (10, 0) -> (10, 54)
  line L11 (-10, 0) -> (-10, 54)
  constraint coincident L4.start L10.start
  constraint coincident L8.end L10.end
  constraint coincident L0.end L11.start
  constraint coincident L9.start L11.end
extrude "Extrude95" add sketch "Sketch62" against normal blind 3 separate body makes body 95
ref_plane "WorkPlane61" through (106.1209, 48.4594, -14) normal (0, 0, -1) x (-0.765705, 0.643192, 0)
sketch "Sketch63" plane through (0, 0, -14) normal (0, 0, -1) x (-1, 0, 0)
  line L0 (-150, 57) -> (150, 57)
  line L1 (150, -3) -> (-150, -3)
  line L2 (-150, 60) -> (150, 60)
  line L3 (150, 57) -> (150, 60)
  line L4 (-150, 57) -> (-150, 60)
  line L5 (150, -6) -> (-150, -6)
  line L6 (-150, -6) -> (-150, -3)
  line L7 (150, -6) -> (150, -3)
  point P0 (-150, 57)
  point P1 (150, 57)
  point P2 (-150, 57)
  point P3 (-150, -3)
  point P4 (150, -3)
  dimension "d732" = -3
  dimension "d733" = -3
  constraint coincident P2 P0
  constraint coincident P1 L0.end
  constraint coincident P4 L1.start
  constraint coincident P3 L1.end
  constraint horizontal L1
  constraint perpendicular L2 L3
  constraint perpendicular L2 L4
  constraint perpendicular L1 L6
  constraint perpendicular L1 L7
extrude "Extrude96" add sketch "Sketch63" along normal blind 6 separate body contours L0 L2 L3 L4 makes body 96
extrude "Extrude97" add sketch "Sketch63" along normal blind 6 separate body contours L1 L5 L6 L7 makes body 97
ref_plane "WorkPlane62" through (0, 58.5, -20) normal (0, 0, -1) x (-1, 0, 0)